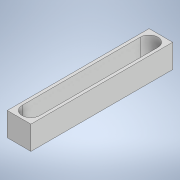
# Autodesk Inventor part: 零件4
Saved by Autodesk Inventor 2022 (Build 260153000, 153)
## iProperties
Created: 2023-03-09
Part Number: 零件4
Material: 一般
Document SubType Name: Modeling
Designer: JOU
Density: 1 g/cm^3
Appearance: 預設
Author: JOU
Autodesk Inventor part; units mm, degrees
ref_plane "YZ Plane" through (0, 0, 0) normal (1, 0, 0) x (0, 1, 0)
ref_plane "XZ Plane" through (0, 0, 0) normal (0, 1, 0) x (-1, 0, 0)
ref_plane "XY Plane" through (0, 0, 0) normal (0, 0, 1) x (1, 0, 0)
sketch "草圖1" plane through (0, 0, 0) normal (0, 1, 0) x (-1, 0, 0)
  line L0 (5.0747, -9.1412) -> (3.0747, -9.1412)
  line L1 (3.0747, -9.1412) -> (3.0747, -21.1412)
  line L2 (3.0747, -21.1412) -> (5.0747, -21.1412)
  line L3 (5.0747, -21.1412) -> (5.0747, -9.1412)
  arc A0 (4.8247, -10.1412) -> (3.3247, -10.1412) centre (4.0747, -10.1412) ccw
  arc A1 (3.3247, -20.1412) -> (4.8247, -20.1412) centre (4.0747, -20.1412) ccw
  line L4 (4.8247, -10.1412) -> (4.8247, -20.1412)
  line L5 (3.3247, -10.1412) -> (3.3247, -20.1412)
  point P0 (0, 0)
  dimension "d3" = 1.5
  dimension "d4" = 2
  dimension "d5" = 1
  dimension "d6" = 1
  dimension "d7" = 1
  dimension "d8" = 12
  constraints: 12 end point, 4 parallel, 4 point on circle, 4 tangent, 2 centre point, 1 horizontal, 1 perpendicular
  measures "d3" diameter of A0
  measures "d4" distance of L0.start L0.end
  measures "d5" distance from line of L1 A0.centre
  measures "d6" distance from line of L0 A0.centre
  measures "d7" distance from line of L2 A1.centre
  measures "d8" distance of L2.end L0.start
extrude "擠出1" add sketch "草圖1" along normal blind 2
